Autodesk Inventor part; units mm, degrees
(part 2 of 2)
  spline S229 degree 2 poles (48.9042, 0.3817) (48.9464, 0.3509) (49.089, 0.2941) (49.1595, 0.2941) knots 0 0 0 1 2 2 2
  spline S230 degree 2 poles (49.1595, 0.2941) (49.2008, 0.2941) (49.2835, 0.3201) (49.311, 0.35) knots 0 0 0 1 2 2 2
  spline S231 degree 2 poles (49.311, 0.35) (49.3378, 0.38) (49.3661, 0.4513) (49.3661, 0.5056) knots 0 0 0 1 2 2 2
  spline S232 degree 2 poles (49.3661, 0.5056) (49.3661, 0.5599) (49.3345, 0.6304) (49.3062, 0.6507) knots 0 0 0 1 2 2 2
  spline S233 degree 2 poles (49.3062, 0.6507) (49.2778, 0.671) (49.2008, 0.6864) (49.1554, 0.6864) knots 0 0 0 1 2 2 2
  line L352 (49.1554, 0.6864) -> (49.0987, 0.6864)
  line L353 (49.0987, 0.6864) -> (49.0987, 0.7974)
  line L354 (49.0987, 0.7974) -> (49.1433, 0.7974)
  spline S234 degree 2 poles (49.1433, 0.7974) (49.2332, 0.7974) (49.3467, 0.8833) (49.3467, 0.9651) knots 0 0 0 1 2 2 2
  spline S235 degree 2 poles (49.3467, 0.9651) (49.3467, 1.0032) (49.3175, 1.0575) (49.294, 1.0737) knots 0 0 0 1 2 2 2
  spline S236 degree 2 poles (49.294, 1.0737) (49.2689, 1.0907) (49.2073, 1.1045) (49.1725, 1.1045) knots 0 0 0 1 2 2 2
  line L355 (45.2147, 0.2039) -> (44.7269, 0.2039)
  line L356 (44.7269, 0.2039) -> (44.7269, 0.306)
  line L357 (44.7269, 0.306) -> (44.9084, 0.306)
  line L358 (44.9084, 0.306) -> (44.9084, 0.9762)
  line L359 (44.9084, 0.9762) -> (44.7269, 0.9762)
  line L360 (44.7269, 0.9762) -> (44.7269, 1.0677)
  spline S237 degree 2 poles (44.7269, 1.0677) (44.8298, 1.0677) (44.9271, 1.1261) (44.9335, 1.2071) knots 0 0 0 1 2 2 2
  line L361 (44.9335, 1.2071) -> (45.0373, 1.2071)
  line L362 (45.0373, 1.2071) -> (45.0373, 0.306)
  line L363 (45.0373, 0.306) -> (45.2147, 0.306)
  line L364 (45.2147, 0.306) -> (45.2147, 0.2039)
  line L365 (46.0154, 0.2039) -> (45.3987, 0.2039)
  line L366 (45.3987, 0.2039) -> (45.3987, 0.3457)
  spline S238 degree 2 poles (45.3987, 0.3457) (45.4651, 0.4081) (45.5835, 0.524) (45.6402, 0.5864) knots 0 0 0 1 2 2 2
  spline S239 degree 2 poles (45.6402, 0.5864) (45.7545, 0.712) (45.8379, 0.8627) (45.8379, 0.9429) knots 0 0 0 1 2 2 2
  spline S240 degree 2 poles (45.8379, 0.9429) (45.8379, 0.9851) (45.812, 1.0483) (45.7885, 1.0685) knots 0 0 0 1 2 2 2
  spline S241 degree 2 poles (45.7885, 1.0685) (45.765, 1.0888) (45.7034, 1.1091) (45.6661, 1.1091) knots 0 0 0 1 2 2 2
  spline S242 degree 2 poles (45.6661, 1.1091) (45.6305, 1.1091) (45.5575, 1.0912) (45.5243, 1.0775) knots 0 0 0 1 2 2 2
  spline S243 degree 2 poles (45.5243, 1.0775) (45.4959, 1.0661) (45.4433, 1.0337) (45.4271, 1.0224) knots 0 0 0 1 2 2 2
  line L367 (45.4271, 1.0224) -> (45.4198, 1.0224)
  line L368 (45.4198, 1.0224) -> (45.4198, 1.165)
  spline S244 degree 2 poles (45.4198, 1.165) (45.4611, 1.1852) (45.6094, 1.2249) (45.6758, 1.2249) knots 0 0 0 1 2 2 2
  spline S245 degree 2 poles (45.6758, 1.2249) (45.816, 1.2249) (45.9741, 1.0767) (45.9741, 0.9502) knots 0 0 0 1 2 2 2
  spline S246 degree 2 poles (45.9741, 0.9502) (45.9741, 0.8911) (45.9465, 0.7922) (45.9222, 0.7501) knots 0 0 0 1 2 2 2
  spline S247 degree 2 poles (45.9222, 0.7501) (45.8979, 0.7063) (45.8274, 0.6204) (45.7885, 0.5791) knots 0 0 0 1 2 2 2
  spline S248 degree 2 poles (45.7885, 0.5791) (45.7253, 0.5102) (45.5705, 0.3627) (45.5243, 0.3198) knots 0 0 0 1 2 2 2
  line L369 (45.5243, 0.3198) -> (46.0154, 0.3198)
  line L370 (46.0154, 0.3198) -> (46.0154, 0.2039)
  line L371 (41.6659, 0.2263) -> (41.178, 0.2263)
  line L372 (41.178, 0.2263) -> (41.178, 0.3284)
  line L373 (41.178, 0.3284) -> (41.3595, 0.3284)
  line L374 (41.3595, 0.3284) -> (41.3595, 0.9986)
  line L375 (41.3595, 0.9986) -> (41.178, 0.9986)
  line L376 (41.178, 0.9986) -> (41.178, 1.0901)
  spline S249 degree 2 poles (41.178, 1.0901) (41.2809, 1.0901) (41.3782, 1.1485) (41.3847, 1.2295) knots 0 0 0 1 2 2 2
  line L377 (41.3847, 1.2295) -> (41.4884, 1.2295)
  line L378 (41.4884, 1.2295) -> (41.4884, 0.3284)
  line L379 (41.4884, 0.3284) -> (41.6659, 0.3284)
  line L380 (41.6659, 0.3284) -> (41.6659, 0.2263)
  line L381 (42.4163, 0.2263) -> (41.9284, 0.2263)
  line L382 (41.9284, 0.2263) -> (41.9284, 0.3284)
  line L383 (41.9284, 0.3284) -> (42.1099, 0.3284)
  line L384 (42.1099, 0.3284) -> (42.1099, 0.9986)
  line L385 (42.1099, 0.9986) -> (41.9284, 0.9986)
  line L386 (41.9284, 0.9986) -> (41.9284, 1.0901)
  spline S250 degree 2 poles (41.9284, 1.0901) (42.0313, 1.0901) (42.1286, 1.1485) (42.1351, 1.2295) knots 0 0 0 1 2 2 2
  line L387 (42.1351, 1.2295) -> (42.2388, 1.2295)
  line L388 (42.2388, 1.2295) -> (42.2388, 0.3284)
  line L389 (42.2388, 0.3284) -> (42.4163, 0.3284)
  line L390 (42.4163, 0.3284) -> (42.4163, 0.2263)
  line L391 (38.2669, 0.1838) -> (37.7791, 0.1838)
  line L392 (37.7791, 0.1838) -> (37.7791, 0.2859)
  line L393 (37.7791, 0.2859) -> (37.9606, 0.2859)
  line L394 (37.9606, 0.2859) -> (37.9606, 0.9561)
  line L395 (37.9606, 0.9561) -> (37.7791, 0.9561)
  line L396 (37.7791, 0.9561) -> (37.7791, 1.0477)
  spline S251 degree 2 poles (37.7791, 1.0477) (37.882, 1.0477) (37.9792, 1.106) (37.9857, 1.1871) knots 0 0 0 1 2 2 2
  line L397 (37.9857, 1.1871) -> (38.0894, 1.1871)
  line L398 (38.0894, 1.1871) -> (38.0894, 0.2859)
  line L399 (38.0894, 0.2859) -> (38.2669, 0.2859)
  line L400 (38.2669, 0.2859) -> (38.2669, 0.1838)
  spline S252 degree 2 poles (39.0732, 0.6838) (39.0732, 0.4148) (38.9168, 0.1628) (38.7539, 0.1628) knots 0 0 0 1 2 2 2
  spline S253 degree 2 poles (38.7539, 0.1628) (38.5886, 0.1628) (38.4338, 0.4196) (38.4338, 0.683) knots 0 0 0 1 2 2 2
  spline S254 degree 2 poles (38.4338, 0.683) (38.4338, 0.9537) (38.5902, 1.2041) (38.7539, 1.2041) knots 0 0 0 1 2 2 2
  spline S255 degree 2 poles (38.7539, 1.2041) (38.9184, 1.2041) (39.0732, 0.9448) (39.0732, 0.6838) knots 0 0 0 1 2 2 2
  spline S256 degree 2 poles (38.9014, 0.3791) (38.9209, 0.4286) (38.9371, 0.5809) (38.9371, 0.6838) knots 0 0 0 1 2 2 2
  spline S257 degree 2 poles (38.9371, 0.6838) (38.9371, 0.7867) (38.9209, 0.9383) (38.9006, 0.9893) knots 0 0 0 1 2 2 2
  spline S258 degree 2 poles (38.9006, 0.9893) (38.8804, 1.0404) (38.8099, 1.0931) (38.7539, 1.0931) knots 0 0 0 1 2 2 2
  spline S259 degree 2 poles (38.7539, 1.0931) (38.698, 1.0931) (38.6259, 1.0404) (38.6048, 0.9877) knots 0 0 0 1 2 2 2
  spline S260 degree 2 poles (38.6048, 0.9877) (38.5846, 0.9367) (38.57, 0.7811) (38.57, 0.683) knots 0 0 0 1 2 2 2
  spline S261 degree 2 poles (38.57, 0.683) (38.57, 0.5777) (38.583, 0.4367) (38.604, 0.3816) knots 0 0 0 1 2 2 2
  spline S262 degree 2 poles (38.604, 0.3816) (38.6235, 0.3297) (38.6956, 0.2738) (38.7539, 0.2738) knots 0 0 0 1 2 2 2
  spline S263 degree 2 poles (38.7539, 0.2738) (38.809, 0.2738) (38.8812, 0.3265) (38.9014, 0.3791) knots 0 0 0 1 2 2 2
  spline S264 degree 2 poles (34.4389, 0.8934) (34.4389, 0.9704) (34.4891, 1.0984) (34.5329, 1.1446) knots 0 0 0 1 2 2 2
  spline S265 degree 2 poles (34.5329, 1.1446) (34.5742, 1.1892) (34.695, 1.2386) (34.7565, 1.2386) knots 0 0 0 1 2 2 2
  spline S266 degree 2 poles (34.7565, 1.2386) (34.8254, 1.2386) (34.9373, 1.1924) (34.9786, 1.1487) knots 0 0 0 1 2 2 2
  spline S267 degree 2 poles (34.9786, 1.1487) (35.0305, 1.0936) (35.0872, 0.9153) (35.0872, 0.7783) knots 0 0 0 1 2 2 2
  spline S268 degree 2 poles (35.0872, 0.7783) (35.0872, 0.6544) (35.0313, 0.4323) (34.977, 0.3586) knots 0 0 0 1 2 2 2
  spline S269 degree 2 poles (34.977, 0.3586) (34.9194, 0.2808) (34.7574, 0.1989) (34.639, 0.1989) knots 0 0 0 1 2 2 2
  spline S270 degree 2 poles (34.639, 0.1989) (34.6123, 0.1989) (34.5515, 0.2046) (34.5256, 0.2127) knots 0 0 0 1 2 2 2
  line L401 (34.5256, 0.2127) -> (34.5256, 0.3416)
  line L402 (34.5256, 0.3416) -> (34.5321, 0.3416)
  spline S271 degree 2 poles (34.5321, 0.3416) (34.5491, 0.3318) (34.6204, 0.3148) (34.6569, 0.3148) knots 0 0 0 1 2 2 2
  spline S272 degree 2 poles (34.6569, 0.3148) (34.7882, 0.3148) (34.9381, 0.4882) (34.9486, 0.6487) knots 0 0 0 1 2 2 2
  spline S273 degree 2 poles (34.9486, 0.6487) (34.8951, 0.6122) (34.7979, 0.579) (34.7403, 0.579) knots 0 0 0 1 2 2 2
  spline S274 degree 2 poles (34.7403, 0.579) (34.6852, 0.579) (34.5937, 0.6033) (34.5475, 0.6381) knots 0 0 0 1 2 2 2
  spline S275 degree 2 poles (34.5475, 0.6381) (34.494, 0.6795) (34.4389, 0.8051) (34.4389, 0.8934) knots 0 0 0 1 2 2 2
  spline S276 degree 2 poles (34.9518, 0.8083) (34.9518, 0.9096) (34.9146, 1.0377) (34.8813, 1.0725) knots 0 0 0 1 2 2 2
  spline S277 degree 2 poles (34.8813, 1.0725) (34.8522, 1.1049) (34.7914, 1.1292) (34.7557, 1.1292) knots 0 0 0 1 2 2 2
  spline S278 degree 2 poles (34.7557, 1.1292) (34.6731, 1.1292) (34.575, 1.0109) (34.575, 0.8991) knots 0 0 0 1 2 2 2
  spline S279 degree 2 poles (34.575, 0.8991) (34.575, 0.8359) (34.6074, 0.754) (34.6431, 0.7249) knots 0 0 0 1 2 2 2
  spline S280 degree 2 poles (34.6431, 0.7249) (34.669, 0.7038) (34.733, 0.69) (34.7703, 0.69) knots 0 0 0 1 2 2 2
  spline S281 degree 2 poles (34.7703, 0.69) (34.8133, 0.69) (34.9121, 0.72) (34.9494, 0.7451) knots 0 0 0 1 2 2 2
  spline S282 degree 2 poles (34.9494, 0.7451) (34.9502, 0.7548) (34.9518, 0.7881) (34.9518, 0.8083) knots 0 0 0 1 2 2 2
  spline S283 degree 2 poles (31.2948, 0.2278) (31.2202, 0.2278) (31.0979, 0.2724) (31.0549, 0.3137) knots 0 0 0 1 2 2 2
  spline S284 degree 2 poles (31.0549, 0.3137) (31.0128, 0.3542) (30.969, 0.4644) (30.969, 0.5268) knots 0 0 0 1 2 2 2
  spline S285 degree 2 poles (30.969, 0.5268) (30.969, 0.6079) (31.0557, 0.744) (31.1384, 0.7845) knots 0 0 0 1 2 2 2
  line L403 (31.1384, 0.7845) -> (31.1384, 0.7886)
  spline S286 degree 2 poles (31.1384, 0.7886) (31.0646, 0.8315) (30.9933, 0.9336) (30.9933, 1.0098) knots 0 0 0 1 2 2 2
  spline S287 degree 2 poles (30.9933, 1.0098) (30.9933, 1.1225) (31.1635, 1.2732) (31.2948, 1.2732) knots 0 0 0 1 2 2 2
  spline S288 degree 2 poles (31.2948, 1.2732) (31.4309, 1.2732) (31.5954, 1.1306) (31.5954, 1.0187) knots 0 0 0 1 2 2 2
  spline S289 degree 2 poles (31.5954, 1.0187) (31.5954, 0.9515) (31.5168, 0.8202) (31.4431, 0.7829) knots 0 0 0 1 2 2 2
  line L404 (31.4431, 0.7829) -> (31.4431, 0.7789)
  spline S290 degree 2 poles (31.4431, 0.7789) (31.5306, 0.7383) (31.6206, 0.6216) (31.6206, 0.5293) knots 0 0 0 1 2 2 2
  spline S291 degree 2 poles (31.6206, 0.5293) (31.6206, 0.4012) (31.4342, 0.2278) (31.2948, 0.2278) knots 0 0 0 1 2 2 2
  spline S292 degree 2 poles (31.4828, 0.5163) (31.4828, 0.5779) (31.4342, 0.6508) (31.3653, 0.6881) knots 0 0 0 1 2 2 2
  spline S293 degree 2 poles (31.3653, 0.6881) (31.3426, 0.7011) (31.2664, 0.731) (31.2186, 0.7505) knots 0 0 0 1 2 2 2
  spline S294 degree 2 poles (31.2186, 0.7505) (31.1635, 0.714) (31.1043, 0.6054) (31.1043, 0.5366) knots 0 0 0 1 2 2 2
  spline S295 degree 2 poles (31.1043, 0.5366) (31.1043, 0.4458) (31.2137, 0.3275) (31.2964, 0.3275) knots 0 0 0 1 2 2 2
  spline S296 degree 2 poles (31.2964, 0.3275) (31.3807, 0.3275) (31.4828, 0.4288) (31.4828, 0.5163) knots 0 0 0 1 2 2 2
  spline S297 degree 2 poles (31.4642, 1.0171) (31.4642, 1.0844) (31.3742, 1.1743) (31.294, 1.1743) knots 0 0 0 1 2 2 2
  spline S298 degree 2 poles (31.294, 1.1743) (31.221, 1.1743) (31.1278, 1.0941) (31.1278, 1.0252) knots 0 0 0 1 2 2 2
  spline S299 degree 2 poles (31.1278, 1.0252) (31.1278, 0.9758) (31.1757, 0.9069) (31.2235, 0.8793) knots 0 0 0 1 2 2 2
  spline S300 degree 2 poles (31.2235, 0.8793) (31.2437, 0.868) (31.3296, 0.8283) (31.3645, 0.8169) knots 0 0 0 1 2 2 2
  spline S301 degree 2 poles (31.3645, 0.8169) (31.4228, 0.8615) (31.4642, 0.9563) (31.4642, 1.0171) knots 0 0 0 1 2 2 2
  line L405 (28.0867, 1.1128) -> (27.6539, 0.2627)
  line L406 (27.6539, 0.2627) -> (27.5113, 0.2627)
  line L407 (27.5113, 0.2627) -> (27.9683, 1.1452)
  line L408 (27.9683, 1.1452) -> (27.4521, 1.1452)
  line L409 (27.4521, 1.1452) -> (27.4521, 1.2627)
  line L410 (27.4521, 1.2627) -> (28.0867, 1.2627)
  line L411 (28.0867, 1.2627) -> (28.0867, 1.1128)
  spline S302 degree 2 poles (24.6318, 0.5428) (24.6318, 0.4658) (24.5807, 0.3354) (24.5378, 0.2916) knots 0 0 0 1 2 2 2
  spline S303 degree 2 poles (24.5378, 0.2916) (24.4932, 0.2454) (24.3814, 0.1976) (24.3141, 0.1976) knots 0 0 0 1 2 2 2
  spline S304 degree 2 poles (24.3141, 0.1976) (24.2469, 0.1976) (24.1358, 0.243) (24.0937, 0.2884) knots 0 0 0 1 2 2 2
  spline S305 degree 2 poles (24.0937, 0.2884) (24.0418, 0.3427) (23.9835, 0.525) (23.9835, 0.6579) knots 0 0 0 1 2 2 2
  spline S306 degree 2 poles (23.9835, 0.6579) (23.9835, 0.7884) (24.037, 0.9983) (24.0929, 1.0761) knots 0 0 0 1 2 2 2
  spline S307 degree 2 poles (24.0929, 1.0761) (24.1472, 1.1522) (24.319, 1.2373) (24.4316, 1.2373) knots 0 0 0 1 2 2 2
  spline S308 degree 2 poles (24.4316, 1.2373) (24.4649, 1.2373) (24.5232, 1.2308) (24.5451, 1.2235) knots 0 0 0 1 2 2 2
  line L412 (24.5451, 1.2235) -> (24.5451, 1.0947)
  line L413 (24.5451, 1.0947) -> (24.5394, 1.0947)
  spline S309 degree 2 poles (24.5394, 1.0947) (24.5208, 1.1044) (24.4527, 1.1214) (24.4138, 1.1214) knots 0 0 0 1 2 2 2
  spline S310 degree 2 poles (24.4138, 1.1214) (24.289, 1.1214) (24.1358, 0.9529) (24.1213, 0.7876) knots 0 0 0 1 2 2 2
  spline S311 degree 2 poles (24.1213, 0.7876) (24.1691, 0.8208) (24.2696, 0.8573) (24.3295, 0.8573) knots 0 0 0 1 2 2 2
  spline S312 degree 2 poles (24.3295, 0.8573) (24.3879, 0.8573) (24.4754, 0.8338) (24.5232, 0.7981) knots 0 0 0 1 2 2 2
  spline S313 degree 2 poles (24.5232, 0.7981) (24.5783, 0.7568) (24.6318, 0.6287) (24.6318, 0.5428) knots 0 0 0 1 2 2 2
  spline S314 degree 2 poles (24.4956, 0.5372) (24.4956, 0.5987) (24.4632, 0.6822) (24.4276, 0.7114) knots 0 0 0 1 2 2 2
  spline S315 degree 2 poles (24.4276, 0.7114) (24.4008, 0.7325) (24.3344, 0.7462) (24.2995, 0.7462) knots 0 0 0 1 2 2 2
  spline S316 degree 2 poles (24.2995, 0.7462) (24.2525, 0.7462) (24.1642, 0.7179) (24.1213, 0.6911) knots 0 0 0 1 2 2 2
  spline S317 degree 2 poles (24.1213, 0.6911) (24.1204, 0.6765) (24.1188, 0.649) (24.1188, 0.6279) knots 0 0 0 1 2 2 2
  spline S318 degree 2 poles (24.1188, 0.6279) (24.1188, 0.5242) (24.1593, 0.397) (24.1901, 0.3637) knots 0 0 0 1 2 2 2
  spline S319 degree 2 poles (24.1901, 0.3637) (24.2185, 0.3321) (24.2801, 0.307) (24.3149, 0.307) knots 0 0 0 1 2 2 2
  spline S320 degree 2 poles (24.3149, 0.307) (24.396, 0.307) (24.4956, 0.4221) (24.4956, 0.5372) knots 0 0 0 1 2 2 2
  spline S321 degree 2 poles (21.1019, 0.5446) (21.1019, 0.4724) (21.0558, 0.3493) (21.0136, 0.3039) knots 0 0 0 1 2 2 2
  spline S322 degree 2 poles (21.0136, 0.3039) (20.9715, 0.2585) (20.8459, 0.2058) (20.7681, 0.2058) knots 0 0 0 1 2 2 2
  spline S323 degree 2 poles (20.7681, 0.2058) (20.6968, 0.2058) (20.5574, 0.2374) (20.5063, 0.2625) knots 0 0 0 1 2 2 2
  line L414 (20.5063, 0.2625) -> (20.5063, 0.4044)
  line L415 (20.5063, 0.4044) -> (20.516, 0.4044)
  spline S324 degree 2 poles (20.516, 0.4044) (20.5314, 0.393) (20.589, 0.3638) (20.6238, 0.3509) knots 0 0 0 1 2 2 2
  spline S325 degree 2 poles (20.6238, 0.3509) (20.6635, 0.3371) (20.7292, 0.3217) (20.7705, 0.3217) knots 0 0 0 1 2 2 2
  spline S326 degree 2 poles (20.7705, 0.3217) (20.811, 0.3217) (20.8872, 0.3509) (20.9148, 0.3825) knots 0 0 0 1 2 2 2
  spline S327 degree 2 poles (20.9148, 0.3825) (20.9399, 0.4125) (20.9658, 0.4919) (20.9658, 0.5454) knots 0 0 0 1 2 2 2
  spline S328 degree 2 poles (20.9658, 0.5454) (20.9658, 0.5989) (20.9366, 0.6669) (20.9091, 0.6896) knots 0 0 0 1 2 2 2
  spline S329 degree 2 poles (20.9091, 0.6896) (20.8807, 0.7147) (20.7964, 0.7358) (20.7454, 0.7358) knots 0 0 0 1 2 2 2
  spline S330 degree 2 poles (20.7454, 0.7358) (20.6903, 0.7358) (20.5809, 0.7188) (20.5477, 0.7115) knots 0 0 0 1 2 2 2
  line L416 (20.5477, 0.7115) -> (20.5477, 1.2269)
  line L417 (20.5477, 1.2269) -> (21.0963, 1.2269)
  line L418 (21.0963, 1.2269) -> (21.0963, 1.1094)
  line L419 (21.0963, 1.1094) -> (20.6765, 1.1094)
  line L420 (20.6765, 1.1094) -> (20.6765, 0.8428)
  spline S331 degree 2 poles (20.6765, 0.8428) (20.7008, 0.846) (20.7478, 0.8484) (20.7673, 0.8484) knots 0 0 0 1 2 2 2
  spline S332 degree 2 poles (20.7673, 0.8484) (20.8443, 0.8484) (20.9504, 0.8233) (20.999, 0.786) knots 0 0 0 1 2 2 2
  spline S333 degree 2 poles (20.999, 0.786) (21.0485, 0.7488) (21.1019, 0.6353) (21.1019, 0.5446) knots 0 0 0 1 2 2 2
  line L421 (17.6503, 0.575) -> (17.5312, 0.575)
  line L422 (17.5312, 0.575) -> (17.5312, 0.2315)
  line L423 (17.5312, 0.2315) -> (17.4023, 0.2315)
  line L424 (17.4023, 0.2315) -> (17.4023, 0.575)
  line L425 (17.4023, 0.575) -> (16.9607, 0.575)
  line L426 (16.9607, 0.575) -> (16.9607, 0.7161)
  line L427 (16.9607, 0.7161) -> (17.408, 1.2315)
  line L428 (17.408, 1.2315) -> (17.5312, 1.2315)
  line L429 (17.5312, 1.2315) -> (17.5312, 0.6828)
  line L430 (17.5312, 0.6828) -> (17.6503, 0.6828)
  line L431 (17.6503, 0.6828) -> (17.6503, 0.575)
  line L432 (17.4023, 0.6828) -> (17.4023, 1.0734)
  line L433 (17.4023, 1.0734) -> (17.066, 0.6828)
  line L434 (17.066, 0.6828) -> (17.4023, 0.6828)
  spline S334 degree 2 poles (13.8028, 1.1051) (13.7663, 1.1051) (13.6942, 1.0873) (13.6594, 1.0735) knots 0 0 0 1 2 2 2
  spline S335 degree 2 poles (13.6594, 1.0735) (13.627, 1.0598) (13.5792, 1.0306) (13.5605, 1.0176) knots 0 0 0 1 2 2 2
  line L435 (13.5605, 1.0176) -> (13.5524, 1.0176)
  line L436 (13.5524, 1.0176) -> (13.5524, 1.1594)
  spline S336 degree 2 poles (13.5524, 1.1594) (13.5962, 1.1829) (13.7461, 1.221) (13.8133, 1.221) knots 0 0 0 1 2 2 2
  spline S337 degree 2 poles (13.8133, 1.221) (13.8814, 1.221) (13.9827, 1.1935) (14.024, 1.1643) knots 0 0 0 1 2 2 2
  spline S338 degree 2 poles (14.024, 1.1643) (14.0678, 1.1327) (14.1132, 1.0411) (14.1132, 0.9795) knots 0 0 0 1 2 2 2
  spline S339 degree 2 poles (14.1132, 0.9795) (14.1132, 0.8969) (14.0046, 0.7721) (13.9284, 0.7559) knots 0 0 0 1 2 2 2
  line L437 (13.9284, 0.7559) -> (13.9284, 0.7461)
  spline S340 degree 2 poles (13.9284, 0.7461) (13.96, 0.7397) (14.0321, 0.7105) (14.0629, 0.6813) knots 0 0 0 1 2 2 2
  spline S341 degree 2 poles (14.0629, 0.6813) (14.0937, 0.6529) (14.1326, 0.5622) (14.1326, 0.4965) knots 0 0 0 1 2 2 2
  spline S342 degree 2 poles (14.1326, 0.4965) (14.1326, 0.4293) (14.0864, 0.315) (14.0443, 0.2713) knots 0 0 0 1 2 2 2
  spline S343 degree 2 poles (14.0443, 0.2713) (14.0005, 0.2259) (13.8766, 0.1789) (13.798, 0.1789) knots 0 0 0 1 2 2 2
  spline S344 degree 2 poles (13.798, 0.1789) (13.7226, 0.1789) (13.5751, 0.2153) (13.5249, 0.2405) knots 0 0 0 1 2 2 2
  line L438 (13.5249, 0.2405) -> (13.5249, 0.3823)
  line L439 (13.5249, 0.3823) -> (13.5346, 0.3823)
  spline S345 degree 2 poles (13.5346, 0.3823) (13.5767, 0.3515) (13.7193, 0.2948) (13.7898, 0.2948) knots 0 0 0 1 2 2 2
  spline S346 degree 2 poles (13.7898, 0.2948) (13.8312, 0.2948) (13.9138, 0.3207) (13.9414, 0.3507) knots 0 0 0 1 2 2 2
  spline S347 degree 2 poles (13.9414, 0.3507) (13.9681, 0.3807) (13.9965, 0.452) (13.9965, 0.5063) knots 0 0 0 1 2 2 2
  spline S348 degree 2 poles (13.9965, 0.5063) (13.9965, 0.5606) (13.9649, 0.6311) (13.9365, 0.6513) knots 0 0 0 1 2 2 2
  spline S349 degree 2 poles (13.9365, 0.6513) (13.9082, 0.6716) (13.8312, 0.687) (13.7858, 0.687) knots 0 0 0 1 2 2 2
  line L440 (13.7858, 0.687) -> (13.7291, 0.687)
  line L441 (13.7291, 0.687) -> (13.7291, 0.798)
  line L442 (13.7291, 0.798) -> (13.7736, 0.798)
  spline S350 degree 2 poles (13.7736, 0.798) (13.8636, 0.798) (13.977, 0.8839) (13.977, 0.9658) knots 0 0 0 1 2 2 2
  spline S351 degree 2 poles (13.977, 0.9658) (13.977, 1.0038) (13.9479, 1.0581) (13.9244, 1.0743) knots 0 0 0 1 2 2 2
  spline S352 degree 2 poles (13.9244, 1.0743) (13.8992, 1.0914) (13.8377, 1.1051) (13.8028, 1.1051) knots 0 0 0 1 2 2 2
  line L443 (10.5858, 0.2195) -> (9.9691, 0.2195)
  line L444 (9.9691, 0.2195) -> (9.9691, 0.3613)
  spline S353 degree 2 poles (9.9691, 0.3613) (10.0355, 0.4237) (10.1538, 0.5396) (10.2106, 0.602) knots 0 0 0 1 2 2 2
  spline S354 degree 2 poles (10.2106, 0.602) (10.3248, 0.7276) (10.4083, 0.8783) (10.4083, 0.9586) knots 0 0 0 1 2 2 2
  spline S355 degree 2 poles (10.4083, 0.9586) (10.4083, 1.0007) (10.3824, 1.0639) (10.3589, 1.0842) knots 0 0 0 1 2 2 2
  spline S356 degree 2 poles (10.3589, 1.0842) (10.3354, 1.1044) (10.2738, 1.1247) (10.2365, 1.1247) knots 0 0 0 1 2 2 2
  spline S357 degree 2 poles (10.2365, 1.1247) (10.2008, 1.1247) (10.1279, 1.1069) (10.0947, 1.0931) knots 0 0 0 1 2 2 2
  spline S358 degree 2 poles (10.0947, 1.0931) (10.0663, 1.0817) (10.0137, 1.0493) (9.9974, 1.038) knots 0 0 0 1 2 2 2
  line L445 (9.9974, 1.038) -> (9.9901, 1.038)
  line L446 (9.9901, 1.038) -> (9.9901, 1.1806)
  spline S359 degree 2 poles (9.9901, 1.1806) (10.0315, 1.2009) (10.1798, 1.2406) (10.2462, 1.2406) knots 0 0 0 1 2 2 2
  spline S360 degree 2 poles (10.2462, 1.2406) (10.3864, 1.2406) (10.5444, 1.0923) (10.5444, 0.9659) knots 0 0 0 1 2 2 2
  spline S361 degree 2 poles (10.5444, 0.9659) (10.5444, 0.9067) (10.5169, 0.8078) (10.4926, 0.7657) knots 0 0 0 1 2 2 2
  spline S362 degree 2 poles (10.4926, 0.7657) (10.4683, 0.7219) (10.3978, 0.636) (10.3589, 0.5947) knots 0 0 0 1 2 2 2
  spline S363 degree 2 poles (10.3589, 0.5947) (10.2957, 0.5258) (10.1409, 0.3783) (10.0947, 0.3354) knots 0 0 0 1 2 2 2
  line L447 (10.0947, 0.3354) -> (10.5858, 0.3354)
  line L448 (10.5858, 0.3354) -> (10.5858, 0.2195)
  line L449 (6.2771, 0.2002) -> (6.2771, 1.0818)
  line L450 (6.2771, 1.0818) -> (5.9416, 1.0818)
  line L451 (5.9416, 1.0818) -> (5.9416, 1.2002)
  line L452 (5.9416, 1.2002) -> (6.7455, 1.2002)
  line L453 (6.7455, 1.2002) -> (6.7455, 1.0818)
  line L454 (6.7455, 1.0818) -> (6.41, 1.0818)
  line L455 (6.41, 1.0818) -> (6.41, 0.2002)
  line L456 (6.41, 0.2002) -> (6.2771, 0.2002)
  line L457 (7.5381, 0.2002) -> (7.3857, 0.2002)
  line L458 (7.3857, 0.2002) -> (7.1426, 0.5989)
  line L459 (7.1426, 0.5989) -> (6.8946, 0.2002)
  line L460 (6.8946, 0.2002) -> (6.7512, 0.2002)
  line L461 (6.7512, 0.2002) -> (7.0697, 0.701)
  line L462 (7.0697, 0.701) -> (6.7609, 1.2002)
  line L463 (6.7609, 1.2002) -> (6.9133, 1.2002)
  line L464 (6.9133, 1.2002) -> (7.1515, 0.8087)
  line L465 (7.1515, 0.8087) -> (7.3946, 1.2002)
  line L466 (7.3946, 1.2002) -> (7.5381, 1.2002)
  line L467 (7.5381, 1.2002) -> (7.2253, 0.7074)
  line L468 (7.2253, 0.7074) -> (7.5381, 0.2002)
  line L469 (3.2987, 0.1897) -> (3.1261, 0.1897)
  line L470 (3.1261, 0.1897) -> (2.8101, 0.5876)
  line L471 (2.8101, 0.5876) -> (2.6577, 0.5876)
  line L472 (2.6577, 0.5876) -> (2.6577, 0.1897)
  line L473 (2.6577, 0.1897) -> (2.5248, 0.1897)
  line L474 (2.5248, 0.1897) -> (2.5248, 1.1897)
  line L475 (2.5248, 1.1897) -> (2.7825, 1.1897)
  spline S364 degree 2 poles (2.7825, 1.1897) (2.8684, 1.1897) (2.9843, 1.1711) (3.037, 1.137) knots 0 0 0 1 2 2 2
  spline S365 degree 2 poles (3.037, 1.137) (3.0897, 1.103) (3.1504, 0.9969) (3.1504, 0.9182) knots 0 0 0 1 2 2 2
  spline S366 degree 2 poles (3.1504, 0.9182) (3.1504, 0.8088) (3.0386, 0.6605) (2.943, 0.6249) knots 0 0 0 1 2 2 2
  line L476 (2.943, 0.6249) -> (3.2987, 0.1897)
  spline S367 degree 2 poles (3.0119, 0.9077) (3.0119, 0.9515) (2.9811, 1.0187) (2.9487, 1.0406) knots 0 0 0 1 2 2 2
  spline S368 degree 2 poles (2.9487, 1.0406) (2.9203, 1.0593) (2.8449, 1.0746) (2.7898, 1.0746) knots 0 0 0 1 2 2 2
  line L477 (2.7898, 1.0746) -> (2.6577, 1.0746)
  line L478 (2.6577, 1.0746) -> (2.6577, 0.6986)
  line L479 (2.6577, 0.6986) -> (2.7744, 0.6986)
  spline S369 degree 2 poles (2.7744, 0.6986) (2.832, 0.6986) (2.9235, 0.7189) (2.9551, 0.7505) knots 0 0 0 1 2 2 2
  spline S370 degree 2 poles (2.9551, 0.7505) (2.9843, 0.7781) (3.0119, 0.8558) (3.0119, 0.9077) knots 0 0 0 1 2 2 2
  line L480 (4.0694, 0.1897) -> (3.9171, 0.1897)
  line L481 (3.9171, 0.1897) -> (3.6739, 0.5884)
  line L482 (3.6739, 0.5884) -> (3.426, 0.1897)
  line L483 (3.426, 0.1897) -> (3.2825, 0.1897)
  line L484 (3.2825, 0.1897) -> (3.601, 0.6905)
  line L485 (3.601, 0.6905) -> (3.2923, 1.1897)
  line L486 (3.2923, 1.1897) -> (3.4446, 1.1897)
  line L487 (3.4446, 1.1897) -> (3.6829, 0.7983)
  line L488 (3.6829, 0.7983) -> (3.926, 1.1897)
  line L489 (3.926, 1.1897) -> (4.0694, 1.1897)
  line L490 (4.0694, 1.1897) -> (3.7566, 0.697)
  line L491 (3.7566, 0.697) -> (4.0694, 0.1897)
  dimension "d0" = 17.2
  dimension "d1" = 66
  dimension "d4" = 3.5
  dimension "d9" = 1.1
  dimension "d10" = 6
  dimension "d11" = 3.3
  dimension "d14" = 3.5
  dimension "d19" = 2.54
  dimension "d20" = 12
  dimension "d21" = 1.54
  dimension "d22" = 0.8
  dimension "d25" = 2.54
  dimension "d28" = 2.54
  dimension "d31" = 4.064
  dimension "d32" = 0.8
  dimension "d35" = 2.54
  dimension "d38" = 2.54
  dimension "d43" = 3.4
  dimension "d44" = 0.2
  dimension "d49" = 2.66
  dimension "d50" = 16.1
  dimension "d51" = 2.66
  constraints: 62 end point, 55 centre point, 23 vertical, 16 point on line, 6 horizontal, 6 parallel, 5 perpendicular, 1 coincident, 193 other
  measures "d0" distance of L0.end L1.end
  measures "d1" distance of L1.end L2.end
  measures "d4" distance of L5.start L6.start
  measures "d9" diameter of A0
  measures "d10" distance between parallel lines of L4 L0
  measures "d11" distance between parallel lines of L5 L3
  measures "d14" distance of A0.centre A1.centre
  measures "d19" distance between parallel lines of L23 L24
  measures "d20" distance between parallel lines of L23 L0
  measures "d21" distance between parallel lines of L25 L3
  measures "d22" diameter of A18
  measures "d25" distance of A18.centre A19.centre
  measures "d28" distance of A18.centre A26.centre
  measures "d31" distance between parallel lines of L26 L27
  measures "d32" diameter of A34
  measures "d35" distance of A34.centre A35.centre
  measures "d38" distance of A34.centre A44.centre
  measures "d43" diameter of A54
  measures "d44" distance between parallel lines of L30 L0
  measures "d49" distance from line of A54.centre L2
  measures "d50" distance from line of A54.centre L1
  measures "d51" distance between parallel lines of L2 L24
extrude "Extrusión1" add sketch "Boceto1" against normal blind 1.6 contours L3 L2 L1 L0 | L111 L112 L113 L114 L115 L116 L117 L118 L119 L120 L121 L122 | S0 S1 S2 S3 L123 L124 S4 S5 S6 L125 L126 S7 S8 | L127 S12 S11 S10 S9 | L128 L129 L130 L131 L132 L133 L134 L135 | S13 S14 S15 S16 L136 L137 S17 S18 S19 L138 L139 S20 S21 | L140 S25 S24 S23 S22 | S26 L141 L142 S27 S28 S29 S30 S31 S32 S33 S34 S35 L143 L144 S36 S37 S38 S39 S40 S41 S42 | S43 L145 L146 S44 S45 S46 S47 S48 S49 S50 S51 L147 L148 S52 S53 S54 S55 S56 S57 S58 | S59 S60 S61 S62 S63 L149 L150 S64 S65 S66 S67 S68 L151 L152 S69 S70 | L153 S71 S72 L154 L155 L156 L157 L158 S73 S74 L159 | S75 S76 S77 S78 L160 L161 S79 S80 S81 L162 L163 S82 S83 | L164 S87 S86 S85 S84 | L165 L166 L167 L168 L169 L170 L171 L172 L173 L174 L175 L176 L177 | S88 L178 L179 S89 S90 S91 S92 S93 S94 S95 S96 L180 L181 S97 S98 S99 S100 S101 S102 S103 | L182 L183 S104 S105 S106 L184 L185 L186 L187 L188 S107 S108 L189 | L190 L191 L192 L193 | L194 L195 L196 L197 | S109 S110 S111 S112 L198 L199 S113 S114 S115 L200 L201 S116 S117 | L202 S121 S120 S119 S118 | L203 L204 L205 L206 | L207 L208 S122 S123 S124 S125 S126 S127 S128 L209 L210 L211 | S132 S131 S130 S129 L212 | L213 L214 L215 L216 L217 L218 L219 | L220 L221 S133 S134 S135 S136 S137 S138 L222 L223 S139 S140 S141 S142 S143 L224 L225 | S144 S145 S146 S147 S148 S149 L226 L227 S150 S151 S152 S153 S154 S155 L228 L229 L230 L231 L232 S156 S157 | L233 L234 L235 L236 L237 L238 L239 L240 L241 L242 | S158 S159 L243 L244 L245 S160 S161 | S165 S164 L248 L247 L246 S163 S162 | S166 S167 S168 S169 S170 S171 L249 L250 S172 S173 S174 S175 S176 S177 L251 L252 L253 L254 L255 S178 S179 | L256 L257 L258 L259 L260 L261 L262 L263 L264 L265 | S180 S181 L266 L267 L268 S182 S183 | S187 S186 L271 L270 L269 S185 S184 | L272 L273 L274 L275 L276 L277 L278 L279 | L282 L281 L280 | L283 L284 L285 L286 L287 L288 L289 S188 S189 S190 L290 | S194 S193 L293 L292 L291 S192 S191 | L294 L295 L296 L297 L298 L299 L300 L301 L302 L303 | L304 L305 L306 L307 L308 L309 L310 L311 L312 L313 | S195 S196 S197 S198 S199 S200 L314 L315 S201 S202 S203 S204 S205 S206 L316 L317 L318 L319 L320 S207 S208 | L321 L322 L323 L324 L325 L326 L327 L328 L329 L330 | S209 S210 L331 L332 L333 S211 S212 | S216 S215 L336 L335 L334 S214 S213 | L337 L338 L339 L340 L341 L342 S217 L343 L344 L345 L346 | S218 S219 L347 L348 S220 S221 S222 S223 L349 S224 S225 S226 S227 S228 L350 L351 S229 S230 S231 S232 S233 L352 L353 L354 S234 S235 S236 | L355 L356 L357 L358 L359 L360 S237 L361 L362 L363 L364 | L365 L366 S238 S239 S240 S241 S242 S243 L367 L368 S244 S245 S246 S247 S248 L369 L370 | L371 L372 L373 L374 L375 L376 S249 L377 L378 L379 L380 | L381 L382 L383 L384 L385 L386 S250 L387 L388 L389 L390 | L391 L392 L393 L394 L395 L396 S251 L397 L398 L399 L400 | S252 S253 S254 S255 | S263 S262 S261 S260 S259 S258 S257 S256 | S264 S265 S266 S267 S268 S269 S270 L401 L402 S271 S272 S273 S274 S275 | S282 S281 S280 S279 S278 S277 S276 | S283 S284 S285 L403 S286 S287 S288 S289 L404 S290 S291 | S296 S295 S294 S293 S292 | S301 S300 S299 S298 S297 | L405 L406 L407 L408 L409 L410 L411 | S302 S303 S304 S305 S306 S307 S308 L412 L413 S309 S310 S311 S312 S313 | S320 S319 S318 S317 S316 S315 S314 | S321 S322 S323 L414 L415 S324 S325 S326 S327 S328 S329 S330 L416 L417 L418 L419 L420 S331 S332 S333 | L421 L422 L423 L424 L425 L426 L427 L428 L429 L430 L431 | L434 L433 L432 | S334 S335 L435 L436 S336 S337 S338 S339 L437 S340 S341 S342 S343 S344 L438 L439 S345 S346 S347 S348 S349 L440 L441 L442 S350 S351 S352 | L443 L444 S353 S354 S355 S356 S357 S358 L445 L446 S359 S360 S361 S362 S363 L447 L448 | L449 L450 L451 L452 L453 L454 L455 L456 | L457 L458 L459 L460 L461 L462 L463 L464 L465 L466 L467 L468 | L469 L484 L476 | L476 L484 L485 L486 L487 L488 L489 L490 L491 L480 L481 L482 L483 | L469 L470 L471 L472 L473 L474 L475 S364 S365 S366 L476 L484 | S370 S369 L479 L478 L477 S368 S367
emboss "Repujado1" sketch "Boceto1" operation add depth 0.1 direction (0, 0, -1) contours L111 L112 L113 L114 L115 L116 L117 L118 L119 L120 L121 L122 | S0 S1 S2 S3 L123 L124 S4 S5 S6 L125 L126 S7 S8 | L128 L129 L130 L131 L132 L133 L134 L135 | S13 S14 S15 S16 L136 L137 S17 S18 S19 L138 L139 S20 S21 | S26 L141 L142 S27 S28 S29 S30 S31 S32 S33 S34 S35 L143 L144 S36 S37 S38 S39 S40 S41 S42 | S43 L145 L146 S44 S45 S46 S47 S48 S49 S50 S51 L147 L148 S52 S53 S54 S55 S56 S57 S58 | S59 S60 S61 S62 S63 L149 L150 S64 S65 S66 S67 S68 L151 L152 S69 S70 | L153 S71 S72 L154 L155 L156 L157 L158 S73 S74 L159 | S75 S76 S77 S78 L160 L161 S79 S80 S81 L162 L163 S82 S83 | L165 L166 L167 L168 L169 L170 L171 L172 L173 L174 L175 L176 L177 | S88 L178 L179 S89 S90 S91 S92 S93 S94 S95 S96 L180 L181 S97 S98 S99 S100 S101 S102 S103 | L182 L183 S104 S105 S106 L184 L185 L186 L187 L188 S107 S108 L189 | L190 L191 L192 L193 | L194 L195 L196 L197 | S109 S110 S111 S112 L198 L199 S113 S114 S115 L200 L201 S116 S117 | L203 L204 L205 L206 | L207 L208 S122 S123 S124 S125 S126 S127 S128 L209 L210 L211 | L213 L214 L215 L216 L217 L218 L219 | L220 L221 S133 S134 S135 S136 S137 S138 L222 L223 S139 S140 S141 S142 S143 L224 L225 | S144 S145 S146 S147 S148 S149 L226 L227 S150 S151 S152 S153 S154 S155 L228 L229 L230 L231 L232 S156 S157 | L233 L234 L235 L236 L237 L238 L239 L240 L241 L242 | S158 S159 L243 L244 L245 S160 S161 | S166 S167 S168 S169 S170 S171 L249 L250 S172 S173 S174 S175 S176 S177 L251 L252 L253 L254 L255 S178 S179 | L256 L257 L258 L259 L260 L261 L262 L263 L264 L265 | S180 S181 L266 L267 L268 S182 S183 | L272 L273 L274 L275 L276 L277 L278 L279 | L283 L284 L285 L286 L287 L288 L289 S188 S189 S190 L290 | L294 L295 L296 L297 L298 L299 L300 L301 L302 L303 | L304 L305 L306 L307 L308 L309 L310 L311 L312 L313 | S195 S196 S197 S198 S199 S200 L314 L315 S201 S202 S203 S204 S205 S206 L316 L317 L318 L319 L320 S207 S208 | L321 L322 L323 L324 L325 L326 L327 L328 L329 L330 | S209 S210 L331 L332 L333 S211 S212 | L337 L338 L339 L340 L341 L342 S217 L343 L344 L345 L346 | S218 S219 L347 L348 S220 S221 S222 S223 L349 S224 S225 S226 S227 S228 L350 L351 S229 S230 S231 S232 S233 L352 L353 L354 S234 S235 S236 | L355 L356 L357 L358 L359 L360 S237 L361 L362 L363 L364 | L365 L366 S238 S239 S240 S241 S242 S243 L367 L368 S244 S245 S246 S247 S248 L369 L370 | L371 L372 L373 L374 L375 L376 S249 L377 L378 L379 L380 | L381 L382 L383 L384 L385 L386 S250 L387 L388 L389 L390 | L391 L392 L393 L394 L395 L396 S251 L397 L398 L399 L400 | S252 S253 S254 S255 | S264 S265 S266 S267 S268 S269 S270 L401 L402 S271 S272 S273 S274 S275 | S283 S284 S285 L403 S286 S287 S288 S289 L404 S290 S291 | L405 L406 L407 L408 L409 L410 L411 | S302 S303 S304 S305 S306 S307 S308 L412 L413 S309 S310 S311 S312 S313 | S321 S322 S323 L414 L415 S324 S325 S326 S327 S328 S329 S330 L416 L417 L418 L419 L420 S331 S332 S333 | L421 L422 L423 L424 L425 L426 L427 L428 L429 L430 L431 | S334 S335 L435 L436 S336 S337 S338 S339 L437 S340 S341 S342 S343 S344 L438 L439 S345 S346 S347 S348 S349 L440 L441 L442 S350 S351 S352 | L443 L444 S353 S354 S355 S356 S357 S358 L445 L446 S359 S360 S361 S362 S363 L447 L448 | L449 L450 L451 L452 L453 L454 L455 L456 | L457 L458 L459 L460 L461 L462 L463 L464 L465 L466 L467 L468 | L469 L484 L476 | L476 L484 L485 L486 L487 L488 L489 L490 L491 L480 L481 L482 L483 | L469 L470 L471 L472 L473 L474 L475 S364 S365 S366 L476 L484
